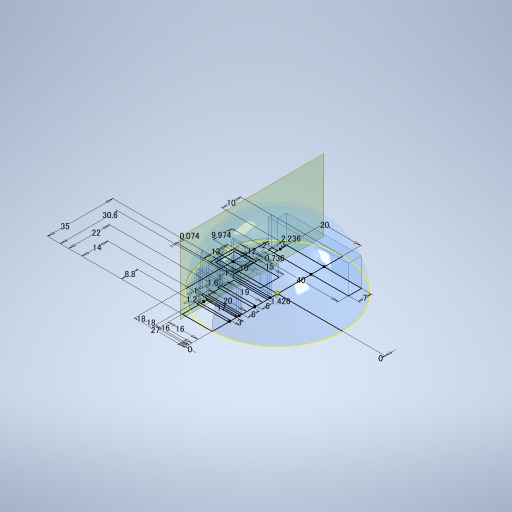
# Autodesk Inventor part: naibu
Saved by Autodesk Inventor 2023 (Build 270158000, 158)
## iProperties
Created: 2022-10-08
Part Number: naibu
Material: 一般
Document SubType Name: Modeling
Designer: ellie
Density: 1 g/cm^3
Appearance: 青 - 光沢
Author: ellie
Autodesk Inventor part; units mm, degrees
ref_plane "YZ Plane" through (0, 0, 0) normal (1, 0, 0) x (0, 1, 0)
ref_plane "XZ Plane" through (0, 0, 0) normal (0, 1, 0) x (-1, 0, 0)
ref_plane "XY Plane" through (0, 0, 0) normal (0, 0, 1) x (1, 0, 0)
sketch "スケッチ1" plane through (0, 0, 0) normal (0, 1, 0) x (-1, 0, 0)
  circle A0 centre (0, 0) radius 35
  line L0 (0, 0) -> (0, -35)
  line L1 (0, 0) -> (0, 35)
  dimension "d0" = 70
  constraints: 4 end point, 2 point on circle, 2 vertical, 1 centre point, 1 coincident
  measures "d0" diameter of A0
revolve "回転1" add sketch "スケッチ1" angle 180 about axis through (0, 0, 0) along (0, 0, 1) picked at (-2.5961, -23.0408) contours L1 L0 A0
sketch "スケッチ5" plane through (0, 0, 0) normal (0, -1, 0) x (1, 0, 0)
  line L0 (-20, -25) -> (20, -25)
  line L1 (20, -25) -> (20, -18)
  line L2 (20, -18) -> (-20, -18)
  line L3 (-20, -18) -> (-20, -25)
  line L4 (-20, -18) -> (-23, -18)
  line L5 (-23, -18) -> (-23, -20)
  line L6 (-23, -20) -> (-20, -20)
  line L7 (-20, -20) -> (-20, -18)
  line L8 (0, 26.2) -> (-17, 26.2)
  line L9 (-17, 26.2) -> (-17, 25)
  line L10 (-17, 25) -> (0, 25)
  line L11 (0, 25) -> (0, 26.2)
  line L12 (0, 21) -> (-20, 21)
  line L13 (-20, 21) -> (-20, 20)
  line L14 (-20, 20) -> (0, 20)
  line L15 (0, 20) -> (0, 21)
  line L16 (0, 13) -> (-19, 13)
  line L17 (-19, 13) -> (-19, 11.4)
  line L18 (-19, 11.4) -> (0, 11.4)
  line L19 (0, 11.4) -> (0, 13)
  line L20 (0, 4.4) -> (-20, 4.4)
  line L21 (-20, 4.4) -> (-20, 3.4)
  line L22 (-20, 3.4) -> (0, 3.4)
  line L23 (0, 3.4) -> (0, 4.4)
  circle A0 centre (0, 0) radius 35 projected
  circle A1 centre (0, 0) radius 35 projected
  line L24 (0, 35) -> (0, -35)
  line L25 (35, 0) -> (-35, 0)
  line L26 (-31.236, 1.9738) -> (-22.236, 1.9738)
  line L27 (-22.236, 1.9738) -> (-22.236, -8.0262)
  line L28 (-22.236, -8.0262) -> (-31.236, -8.0262)
  line L29 (-31.236, -8.0262) -> (-31.236, 1.9738)
  line L30 (-22.236, 1.9738) -> (-7.236, 1.9738)
  line L31 (-7.236, 1.9738) -> (-7.236, -8.0262)
  line L32 (-7.236, -8.0262) -> (-22.236, -8.0262)
  line L33 (-22.236, -8.0262) -> (-22.236, 1.9738)
  line L34 (-27, 22.2711) -> (-27, -22.2711)
  line L35 (-20.736, 3.4738) -> (-32.736, 3.4738)
  line L36 (-32.736, 3.4738) -> (-32.736, -9.5262)
  line L37 (-32.736, -9.5262) -> (-20.736, -9.5262)
  line L38 (-20.736, -9.5262) -> (-20.736, 3.4738)
  line L39 (-20.736, 3.4738) -> (-32.736, -9.5262) construction
  line L40 (-32.736, 3.4738) -> (-20.736, -9.5262) construction
  line L41 (-16, 26.2) -> (0, 26.2)
  line L42 (0, 26.2) -> (0, 35)
  line L43 (0, 35) -> (-16, 35)
  line L44 (-16, 35) -> (-16, 26.2)
  line L45 (-16, 25) -> (0, 25)
  line L46 (0, 25) -> (0, 22)
  line L47 (0, 22) -> (-16, 22)
  line L48 (-16, 22) -> (-16, 25)
  line L49 (-18, 13) -> (0, 13)
  line L50 (0, 13) -> (0, 19)
  line L51 (0, 19) -> (-18, 19)
  line L52 (-18, 19) -> (-18, 13)
  line L53 (-18, 11.4) -> (0, 11.4)
  line L54 (0, 11.4) -> (0, 5.4)
  line L55 (0, 5.4) -> (-18, 5.4)
  line L56 (-18, 5.4) -> (-18, 11.4)
  line L57 (-22.236, -3.0262) -> (-37.4009, -3.0262)
  point P0 (0, -25)
  point P1 (0, -18)
  point P2 (-20, -20)
  point P3 (0, 25.6)
  point P4 (0, 20.5)
  point P5 (0, 12.2)
  point P6 (0, 3.9)
  point P7 (-20, -21.5)
  point P8 (-27, 1.9738)
  point P9 (-27, -8.0262)
  point P10 (-26.736, -3.0262)
  point P11 (-16, 23.5)
  point P12 (-16, 31.1288)
  point P13 (0, 25)
  point P14 (0, 11.4)
  dimension "d12" = 40
  dimension "d13" = 7
  dimension "d21" = 3
  dimension "d22" = 2
  dimension "d23" = 17
  dimension "d24" = 1.2
  dimension "d27" = 20
  dimension "d28" = 1
  dimension "d30" = 19
  dimension "d31" = 1.6
  dimension "d33" = 1
  dimension "d88" = 0
  dimension "d89" = 0
  dimension "d90" = 10
  dimension "d92" = 20
  dimension "d93" = 8.8
  dimension "d94" = 14
  dimension "d95" = 22
  dimension "d96" = 30.6
  dimension "d97" = 9
  dimension "d98" = 10
  dimension "d99" = 1.4262
  dimension "d100" = 2.236
  dimension "d101" = 15
  dimension "d102" = 9.9738
  dimension "d113" = 27
  dimension "d116" = 12
  dimension "d117" = 13
  dimension "d120" = 0.0738
  dimension "d121" = 0.736
  dimension "d122" = 16
  dimension "d123" = 35
  dimension "d124" = 3
  dimension "d125" = 16
  dimension "d126" = 6
  dimension "d127" = 6
  dimension "d128" = 18
  dimension "d129" = 18
  constraints: 114 end point, 26 parallel, 15 horizontal, 13 perpendicular, 11 midpoint, 4 point on line, 1 vertical, 18 other
  measures "d12" distance of L2.end L1.end
  measures "d13" distance of L1.end L0.end
  measures "d21" distance of L6.end L5.end
  measures "d22" distance of L5.end L4.end
  measures "d23" distance of L10.end L9.end
  measures "d24" distance of L9.end L8.end
  measures "d27" distance of L14.end L13.end
  measures "d28" distance of L13.end L12.end
  measures "d30" distance of L18.end L17.end
  measures "d31" distance of L17.end L16.end
  measures "d33" distance of L21.end L20.end
  measures "d89" distance from line of point (0, 0) L25
  measures "d90" distance from line of L0 point (0, -35)
  measures "d92" distance of the line from the sketch origin of L3
  measures "d93" distance from line of L8 point (0, 35)
  measures "d94" distance from line of L12 point (0, 35)
  measures "d95" distance from line of L16 point (0, 35)
  measures "d96" distance from line of L20 point (0, 35)
  measures "d97" distance of L27.end L28.end
  measures "d98" distance of L26.end L27.end
  measures "d99" distance between parallel lines of L26 L22
  measures "d100" horizontal distance of L57.start point (-20, -21.5)
  measures "d101" distance of L31.end L32.end
  measures "d102" distance between parallel lines of L32 L2
  measures "d113" distance of the line from the sketch origin of L34
  measures "d116" distance of L37.end L36.end
  measures "d117" distance of L36.end L35.end
  measures "d120" distance between parallel lines of L35 L22
  measures "d121" distance between parallel lines of L3 L38
  measures "d122" distance of the line from the sketch origin of L44
  measures "d123" distance between parallel lines of L43 L25
  measures "d124" distance of L45.end L46.end
  measures "d126" distance of L50.end L49.end
  measures "d127" distance of L53.end L54.end
  measures "d128" distance of the line from the sketch origin of L56
  measures "d129" distance of the line from the sketch origin of L52
extrude "GNSボード" cut sketch "スケッチ5" against normal blind 16 contours L11 L10 L9 L8
extrude "GNSボード止めるよう" cut sketch "スケッチ5" against normal blind 15 contours L24 L8 L44 A0 | L24 L47 L48 L10
extrude "アルミ板１" cut sketch "スケッチ5" against normal blind 20 contours L15 L14 L13 L12
extrude "メイン基板" cut sketch "スケッチ5" against normal blind 17.5 contours L18 L17 L16 L19
extrude "メイン止めるよう" cut sketch "スケッチ5" against normal blind 16.5 contours L55 L56 L18 L24 | L16 L52 L51 L24
extrude "アルミ板２" cut sketch "スケッチ5" against normal blind 17.5 contours L22 L21 L20 L23
extrude "モーター" cut sketch "スケッチ5" against normal blind 6 contours L31 L32 L38 L25 | L25 L38 L30 L31 | L38 L32 L27 L25 | L25 L27 L30 L38 | L34 L57 L27 L28 | L28 L29 L57 L34 | L27 L57 L34 L25 | L25 L34 L26 L27 | L29 L25 L34 L57 | L25 L29 L26 L34
extrude "モーター受け" add sketch "スケッチ5" against normal blind 9 contours L37 L36 L57 L29 L28 L34 | L34 L28 L32 L38 L37 | L38 L32 L27 L25 | L25 L27 L30 L38 | L36 L25 L29 L57 | L34 L57 L27 L28 | L28 L29 L57 L34 | L27 L57 L34 L25 | L25 L34 L26 L27 | L30 L26 L34 L35 L38 | L36 L35 L34 L26 L29 L25 | L29 L25 L34 L57 | L25 L29 L26 L34
extrude "電池ボックス入れ" cut sketch "スケッチ5" against normal blind 15 contours L3 L2 L24 L0 | L24 L2 L1 L0 | L6 L5 L4 L3
extrude "サイドかっと" cut sketch "スケッチ5" against normal blind 1 contours A0 L57 L36 L37 L34 | A0 L25 L36 L57 | L37 L36 L57 L29 L28 L34 | A0 L34 L35 L36 L25 | L36 L25 L29 L57 | L36 L35 L34 L26 L29 L25
ref_plane "作業平面3" through (-32.736, 9, -9.5262) normal (-1, 0, 0) x (0, 0, -1)
sketch "スケッチ23" plane through (-32.736, 9, -9.5262) normal (-1, 0, 0) x (0, 0, -1)
  line L0 (-11.5, 9) -> (-1.5, 9) projected
  circle A0 centre (-6.5, 9) radius 2.5
  point P0 (-9.5262, 9)
  dimension "d134" = 5
  constraints: 1 centre point, 1 midpoint
  measures "d134" diameter of A0
extrude "押し出し21" cut sketch "スケッチ23" against normal blind 2
